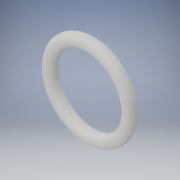
# Autodesk Inventor part: joint
Saved by Autodesk Inventor 2019 (Build 230136000, 136)
## iProperties
Created: 2018-05-05
Part Number: joint
Material: Générique
Document SubType Name: Modeling
Designer: Theo
Density: 1 g/cm^3
Appearance: Par défaut
Author: Theo
Autodesk Inventor part; units mm, degrees
ref_plane "YZ Plane" through (0, 0, 0) normal (1, 0, 0) x (0, 1, 0)
ref_plane "XZ Plane" through (0, 0, 0) normal (0, 1, 0) x (-1, 0, 0)
ref_plane "XY Plane" through (0, 0, 0) normal (0, 0, 1) x (1, 0, 0)
sketch "Esquisse1" plane through (0, 0, 0) normal (1, 0, 0) x (0, 1, 0)
  circle A0 centre (13.5, -2) radius 2
  line L0 (0, 0) -> (0, -15.8798)
  point P0 (13.5, 0)
  point P1 (11.5, -2)
  dimension "d0" = 4
  dimension "d2" = 23
  constraints: 2 end point, 2 horizontal alignment, 2 point on circle, 1 centre point, 1 vertical, 1 vertical alignment
  measures "d0" diameter of A0
  measures "d2" diameter of A0.end L0
revolve "Révolution1" add sketch "Esquisse1" angle 360 about axis through (0, 0, 0) along (0, 0, -1)
